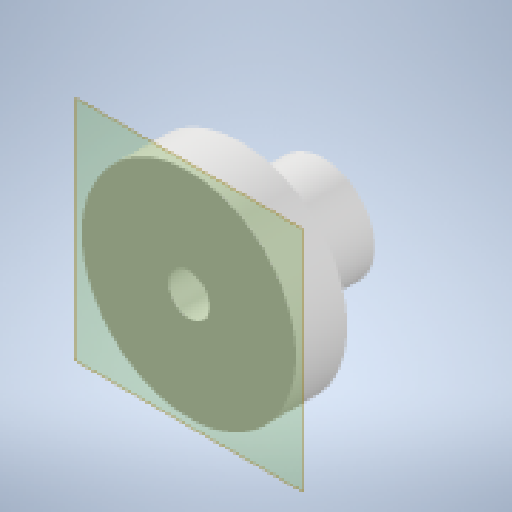
# Autodesk Inventor part: uchwytna wal
Saved by Autodesk Inventor 2023 (Build 270158000, 158)
## iProperties
Created: 2023-06-03
Part Number: uchwytna wal
Material: Ogólny
Document SubType Name: Modeling
Designer: Kamil
Density: 1 g/cm^3
Appearance: Domyślna
Author: Kamil
Autodesk Inventor part; units mm, degrees
ref_plane "YZ Plane" through (0, 0, 0) normal (1, 0, 0) x (0, 1, 0)
ref_plane "XZ Plane" through (0, 0, 0) normal (0, 1, 0) x (-1, 0, 0)
ref_plane "XY Plane" through (0, 0, 0) normal (0, 0, 1) x (1, 0, 0)
ref_plane "Płaszczyzna konstrukcyjna1" through (19.4174, -17.0771, -1.3913) normal (0, 0, -1) x (-1, 0, 0)
sketch "Szkic1" plane through (19.4174, -17.0771, -1.3913) normal (0, 0, -1) x (-1, 0, 0)
  circle A0 centre (7.2744, 10.8616) radius 20.7161 projected
  circle A1 centre (7.2744, 10.8616) radius 4
  circle A2 centre (7.2744, 10.8616) radius 7.5
  point P0 (19.4174, 17.0771)
  dimension "d0" = 8
  dimension "d1" = 15
  constraints: 2 centre point, 2 coincident
  measures "d0" diameter of A1
  measures "d1" diameter of A2
extrude "Wyciągnięcie proste1" add sketch "Szkic1" along normal blind 10 contours A0 | A2
sketch "Szkic2" plane through (12.143, -6.2155, -11.3913) normal (0, 0, -1) x (-1, 0, 0)
  circle A0 centre (0, 0) radius 20.7161 projected
  circle A1 centre (0, 0) radius 4 projected
  circle A2 centre (0, 0) radius 4 projected
  circle A3 centre (0, 0) radius 10
  point P0 (12.143, 6.2155)
  dimension "d4" = 20
  constraints: 1 centre point, 1 coincident
  measures "d4" diameter of A3
extrude "Wyciągnięcie proste2" add sketch "Szkic2" along normal blind 16 contours A3
